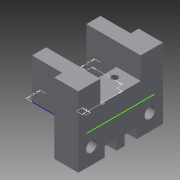
# Autodesk Inventor part: servo_clip_holder1
Saved by Autodesk Inventor 2015 (Build 190159000, 159)
## iProperties
Created: 2017-12-03
Part Number: servo_clip_holder1
Material: Generic
Document SubType Name: Modeling
Designer: Anshul
Density: 1 g/cm^3
Appearance: Default
Author: Anshul
Autodesk Inventor part; units mm, degrees
ref_plane "YZ Plane" through (0, 0, 0) normal (1, 0, 0) x (0, 1, 0)
ref_plane "XZ Plane" through (0, 0, 0) normal (0, 1, 0) x (-1, 0, 0)
ref_plane "XY Plane" through (0, 0, 0) normal (0, 0, 1) x (1, 0, 0)
sketch "Sketch1" plane through (0, 0, 0) normal (0, 1, 0) x (-1, 0, 0)
  line L0 (0, 0) -> (0, -20)
  line L1 (0, -20) -> (15, -20)
  line L2 (15, -20) -> (15, -27)
  line L3 (15, -27) -> (0, -27)
  line L4 (0, 0) -> (15, 0)
  line L5 (15, 0) -> (15, 7)
  line L6 (15, 7) -> (0, 7)
  line L7 (-4, -20) -> (0, -20)
  circle A0 centre (-4, -5) radius 1.6
  circle A1 centre (-4, -15) radius 1.6
  line L8 (0, 7) -> (-12, 7)
  line L9 (-12, 7) -> (-12, -27)
  line L10 (-12, -27) -> (0, -27)
  line L11 (0, -20) -> (-12, -20)
  line L12 (-12, 0) -> (-12, 7)
  line L13 (0, 0) -> (-4, 0)
  line L14 (-4, 0) -> (-12, 0)
  line L15 (15, 0) -> (-12, 0)
  line L16 (0, 7) -> (0, 0)
  line L17 (0, -20) -> (0, -27)
  line L18 (-4, -8) -> (-12, -8)
  line L19 (-4, -8) -> (0, -8)
  line L20 (-4, -2) -> (-12, -2)
  line L21 (-4, -2) -> (0, -2)
  line L22 (-4, -18) -> (0, -18)
  line L23 (-4, -18) -> (-12, -18)
  line L24 (-4, -12) -> (-12, -12)
  line L25 (-4, -12) -> (0, -12)
  dimension "d0" = 20
  dimension "d1" = 15
  dimension "d2" = 7
  dimension "d4" = 7
  dimension "d5" = 4
  constraints: 52 end point, 17 point on line, 13 perpendicular, 4 collinear, 2 centre point, 1 horizontal, 1 vertical
  measures "d0" distance of L0.start L0.end
  measures "d1" distance of L0.end L1.end
  measures "d2" distance of L1.end L2.end
  measures "d4" distance of L4.end L5.end
  measures "d5" distance of L0.start L13.end
extrude "Extrusion1" add sketch "Sketch1" along normal blind 20 contours L16 L6 L5 L4 | L13 L14 L9 L8 L16 | L17 L10 L9 L11 L7 | L1 L2 L3 L17
extrude "Extrusion2" add sketch "Sketch1" along normal blind 9 contours L0 L21 L20 L9 L14 L13 | L0 L19 L18 L9 L20 L21 | L0 L25 L24 L9 L18 L19 | L0 L22 L23 L9 L24 L25 | L0 L7 L11 L9 L23 L22
extrude "Extrusion3" add sketch "Sketch1" against normal blind 15 contours L0 L21 L20 L9 L14 L13 | L13 L14 L9 L8 L16 | L0 L25 L24 L9 L18 L19 | L0 L7 L11 L9 L23 L22 | L17 L10 L9 L11 L7
extrude "Extrusion4" add sketch "Sketch1" against normal blind 10 contours L0 L19 L18 L9 L20 L21 | L0 L22 L23 L9 L24 L25
sketch "Sketch2" plane through (-15, 20, 7) normal (0, 0, 1) x (1, 0, 0)
  line L0 (15, -20) -> (15, 0)
  line L1 (0, 0) -> (27, 0) projected
  line L2 (15, 0) -> (27, 0)
  line L3 (27, 0) -> (27, -35)
  line L4 (27, -35) -> (15, -35)
  line L5 (15, -35) -> (15, -20)
  constraints: 10 end point, 3 perpendicular, 1 collinear, 1 point on line, 1 vertical
extrude "Extrusion5" add sketch "Sketch2" along normal blind 4
sketch "Sketch3" plane through (12, 20, -27) normal (0, 0, -1) x (-1, 0, 0)
  line L0 (0, -35) -> (12, -35)
  line L1 (12, -35) -> (12, 0)
  line L2 (12, 0) -> (0, 0)
  line L3 (27, 0) -> (0, 0) projected
  line L4 (0, 0) -> (0, -35)
  line L5 (0, -35) -> (0, 0) projected
  point P0 (12, -20)
  constraints: 8 end point, 2 collinear, 1 horizontal, 1 perpendicular
extrude "Extrusion6" add sketch "Sketch3" along normal blind 4
sketch "Sketch4" plane through (12, 9, -20) normal (1, 0, 0) x (0, 0, -1)
  line L0 (-31, -24) -> (-18, -24)
  line L1 (-18, -24) -> (-31, -24) projected
  line L2 (-24.5, -24) -> (-24.5, -16)
  line L3 (-2, -24) -> (11, -24)
  line L4 (4.5, -24) -> (4.5, -16)
  circle A0 centre (-24.5, -16) radius 2.65
  circle A1 centre (4.5, -16) radius 2.65
  point P0 (-20, -9)
  dimension "d27" = 8
  dimension "d28" = 8
  dimension "d29" = 5.3
  dimension "d30" = 5.3
  constraints: 8 end point, 2 centre point, 2 coincident, 2 midpoint, 2 vertical, 1 collinear, 1 horizontal
  measures "d27" distance of L2.start L2.end
  measures "d28" distance of L4.start L4.end
  measures "d29" diameter of A0
  measures "d30" diameter of A1
extrude "Extrusion7" cut sketch "Sketch4" against normal blind 13
body "Solid1"
